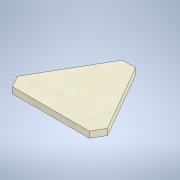
# Autodesk Inventor part: CommandToken_Single
Saved by Autodesk Inventor 2021 (Build 250183000, 183)
## iProperties
Created: 2023-03-16
Part Number: CommandToken_Single
Material: Paper
Document SubType Name: Modeling
Designer: Bradley
Density: 0.93 g/cm^3
Appearance: Cardboard - Chipboard
Author: Bradley
Autodesk Inventor part; units mm, degrees
ref_plane "YZ Plane" through (0, 0, 0) normal (1, 0, 0) x (0, 1, 0)
ref_plane "XZ Plane" through (0, 0, 0) normal (0, 1, 0) x (-1, 0, 0)
ref_plane "XY Plane" through (0, 0, 0) normal (0, 0, 1) x (1, 0, 0)
sketch "Sketch1" plane through (0, 0, 0) normal (0, 1, 0) x (-1, 0, 0)
  line L0 (1.85, -13.4652) -> (-1.85, -13.4652)
  line L1 (-1.85, -13.4652) -> (-12.5862, 5.1305)
  line L2 (-12.5862, 5.1305) -> (-10.7362, 8.3348)
  line L3 (-10.7362, 8.3348) -> (10.7362, 8.3348)
  line L4 (10.7362, 8.3348) -> (12.5862, 5.1305)
  line L5 (12.5862, 5.1305) -> (1.85, -13.4652)
  circle A0 centre (0, 0) radius 8.3348 construction
  dimension "d0" = 21.8
  dimension "d1" = 3.7
  constraints: 12 end point, 4 equal length, 3 parallel, 3 tangent, 1 centre point, 1 coincident, 1 horizontal
  measures "d0" distance between parallel lines of L2 L5
  measures "d1" distance of L0.start L0.end
extrude "Extrusion1" add sketch "Sketch1" along normal mid plane 1.75
body "Solid1"
